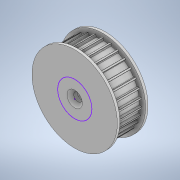
# Autodesk Inventor part: zahnrad
Saved by Autodesk Inventor 2021 (Build 250183000, 183)
## iProperties
Created: 2021-08-02
Part Number: zahnrad
Material: Generisch
Document SubType Name: Modeling
Designer: stroh
Density: 1 g/cm^3
Appearance: Vorgabe
Author: stroh
Autodesk Inventor part; units mm, degrees
ref_plane "YZ Plane" through (0, 0, 0) normal (1, 0, 0) x (0, 1, 0)
ref_plane "XZ Plane" through (0, 0, 0) normal (0, 1, 0) x (-1, 0, 0)
ref_plane "XY Plane" through (0, 0, 0) normal (0, 0, 1) x (1, 0, 0)
sketch "Skizze1" plane through (0, 0, 0) normal (0, 0, 1) x (1, 0, 0)
  line L0 (-32.159, 0) -> (32.1594, 0) projected
  line L1 (0, -33.3687) -> (0, 39.89) projected
  circle A0 centre (0, 0) radius 21.4859
  line L2 (0, 21.3008) -> (0, 29.4245) construction
  line L3 (0.5, 21.4801) -> (-0.5, 21.4801)
  line L4 (-0.4048, 22.9801) -> (0.395, 22.9801)
  line L5 (-0.5, 22.8801) -> (-0.5, 21.4801)
  line L6 (0.395, 22.9801) -> (0.5, 22.8801)
  line L7 (-0.4048, 22.9801) -> (-0.5, 22.8801)
  line L8 (0.5, 22.8801) -> (0.5, 21.4801)
  line L9 (-4.116, 22.5124) -> (-3.8341, 21.141)
  line L10 (-4.239, 22.5892) -> (-4.116, 22.5124)
  line L11 (-5.0223, 22.4282) -> (-4.239, 22.5892)
  line L12 (-5.0223, 22.4282) -> (-5.0955, 22.3111)
  line L13 (-5.0955, 22.3111) -> (-4.8137, 20.9398)
  line L14 (-3.8341, 21.141) -> (-4.8137, 20.9398)
  line L15 (-8.5634, 21.223) -> (-8.0113, 19.9365)
  line L16 (-8.6994, 21.2735) -> (-8.5634, 21.223)
  line L17 (-9.4343, 20.9581) -> (-8.6994, 21.2735)
  line L18 (-9.4343, 20.9581) -> (-9.4824, 20.8287)
  line L19 (-9.4824, 20.8287) -> (-8.9303, 19.5421)
  line L20 (-8.0113, 19.9365) -> (-8.9303, 19.5421)
  line L21 (-12.6603, 19.0648) -> (-11.8605, 17.9157)
  line L22 (-12.8036, 19.0869) -> (-12.6603, 19.0648)
  line L23 (-13.46, 18.63) -> (-12.8036, 19.0869)
  line L24 (-13.46, 18.63) -> (-13.4811, 18.4935)
  line L25 (-13.4811, 18.4935) -> (-12.6813, 17.3444)
  line L26 (-11.8605, 17.9157) -> (-12.6813, 17.3444)
  line L27 (-16.2388, 16.126) -> (-15.2241, 15.1615)
  line L28 (-16.3837, 16.1188) -> (-16.2388, 16.126)
  line L29 (-16.9347, 15.5392) -> (-16.3837, 16.1188)
  line L30 (-16.9347, 15.5392) -> (-16.9278, 15.4012)
  line L31 (-16.9278, 15.4012) -> (-15.9131, 14.4367)
  line L32 (-15.2241, 15.1615) -> (-15.9131, 14.4367)
  line L33 (-19.1526, 12.5271) -> (-17.9645, 11.7865)
  line L34 (-19.293, 12.4908) -> (-19.1526, 12.5271)
  line L35 (-19.716, 11.8121) -> (-19.293, 12.4908)
  line L36 (-19.716, 11.8121) -> (-19.6815, 11.6784)
  line L37 (-19.6815, 11.6784) -> (-18.4934, 10.9379)
  line L38 (-17.9645, 11.7865) -> (-18.4934, 10.9379)
  line L39 (-21.2822, 8.4153) -> (-19.9694, 7.929)
  line L40 (-21.4125, 8.3515) -> (-21.2822, 8.4153)
  line L41 (-21.6902, 7.6015) -> (-21.4125, 8.3515)
  line L42 (-21.6902, 7.6015) -> (-21.6295, 7.4775)
  line L43 (-21.6295, 7.4775) -> (-20.3167, 6.9913)
  line L44 (-19.9694, 7.929) -> (-20.3167, 6.9913)
  line L45 (-22.5405, 3.9589) -> (-21.1567, 3.7469)
  line L46 (-22.6553, 3.8703) -> (-22.5405, 3.9589)
  line L47 (-22.7764, 3.0797) -> (-22.6553, 3.8703)
  line L48 (-22.7764, 3.0797) -> (-22.692, 2.9704)
  line L49 (-22.692, 2.9704) -> (-21.3081, 2.7584)
  line L50 (-21.1567, 3.7469) -> (-21.3081, 2.7584)
  line L51 (-22.8761, -0.6595) -> (-21.4779, -0.5886)
  line L52 (-22.9706, -0.7694) -> (-22.8761, -0.6595)
  line L53 (-22.9301, -1.5682) -> (-22.9706, -0.7694)
  line L54 (-22.9301, -1.5682) -> (-22.8254, -1.6582)
  line L55 (-22.8254, -1.6582) -> (-21.4272, -1.5873)
  line L56 (-21.4779, -0.5886) -> (-21.4272, -1.5873)
  line L57 (-22.275, -5.2509) -> (-20.9197, -4.9)
  line L58 (-22.3455, -5.3776) -> (-22.275, -5.2509)
  line L59 (-22.1451, -6.1519) -> (-22.3455, -5.3776)
  line L60 (-22.1451, -6.1519) -> (-22.0244, -6.219)
  line L61 (-22.0244, -6.219) -> (-20.6691, -5.8681)
  line L62 (-20.9197, -4.9) -> (-20.6691, -5.8681)
  line L63 (-20.7621, -9.6274) -> (-19.5051, -9.0108)
  line L64 (-20.8056, -9.7657) -> (-20.7621, -9.6274)
  line L65 (-20.4534, -10.4837) -> (-20.8056, -9.7657)
  line L66 (-20.4534, -10.4837) -> (-20.3217, -10.5252)
  line L67 (-20.3217, -10.5252) -> (-19.0647, -9.9086)
  line L68 (-19.5051, -9.0108) -> (-19.0647, -9.9086)
  line L69 (-18.3991, -13.6097) -> (-17.292, -12.7527)
  line L70 (-18.4139, -13.7539) -> (-18.3991, -13.6097)
  line L71 (-17.9243, -14.3863) -> (-18.4139, -13.7539)
  line L72 (-17.9243, -14.3863) -> (-17.787, -14.4004)
  line L73 (-17.787, -14.4004) -> (-16.6799, -13.5435)
  line L74 (-17.292, -12.7527) -> (-16.6799, -13.5435)
  line L75 (-15.2828, -17.0348) -> (-14.3709, -15.9725)
  line L76 (-15.2683, -17.1791) -> (-15.2828, -17.0348)
  line L77 (-14.6615, -17.7) -> (-15.2683, -17.1791)
  line L78 (-14.6615, -17.7) -> (-14.5241, -17.6861)
  line L79 (-14.5241, -17.6861) -> (-13.6122, -16.6239)
  line L80 (-14.3709, -15.9725) -> (-13.6122, -16.6239)
  line L81 (-11.5409, -19.7625) -> (-10.8615, -18.5384)
  line L82 (-11.4976, -19.9009) -> (-11.5409, -19.7625)
  line L83 (-10.7984, -20.289) -> (-11.4976, -19.9009)
  line L84 (-10.7984, -20.289) -> (-10.6666, -20.2478)
  line L85 (-10.6666, -20.2478) -> (-9.9872, -19.0237)
  line L86 (-10.8615, -18.5384) -> (-9.9872, -19.0237)
  line L87 (-7.3265, -21.6811) -> (-6.9074, -20.3453)
  line L88 (-7.2563, -21.808) -> (-7.3265, -21.6811)
  line L89 (-6.4932, -22.0474) -> (-7.2563, -21.808)
  line L90 (-6.4932, -22.0474) -> (-6.3724, -21.9805)
  line L91 (-6.3724, -21.9805) -> (-5.9533, -20.6447)
  line L92 (-6.9074, -20.3453) -> (-5.9533, -20.6447)
  line L93 (-2.8122, -22.7121) -> (-2.6705, -21.3193)
  line L94 (-2.7178, -22.8222) -> (-2.8122, -22.7121)
  line L95 (-1.9222, -22.9031) -> (-2.7178, -22.8222)
  line L96 (-1.9222, -22.9031) -> (-1.8173, -22.8133)
  line L97 (-1.8173, -22.8133) -> (-1.6757, -21.4205)
  line L98 (-2.6705, -21.3193) -> (-1.6757, -21.4205)
  line L99 (1.8173, -22.8133) -> (1.6757, -21.4205)
  line L100 (1.9319, -22.9022) -> (1.8173, -22.8133)
  line L101 (2.7276, -22.8212) -> (1.9319, -22.9022)
  line L102 (2.7276, -22.8212) -> (2.8122, -22.7121)
  line L103 (2.8122, -22.7121) -> (2.6705, -21.3193)
  line L104 (1.6757, -21.4205) -> (2.6705, -21.3193)
  line L105 (6.3724, -21.9805) -> (5.9533, -20.6447)
  line L106 (6.5025, -22.0445) -> (6.3724, -21.9805)
  line L107 (7.2656, -21.805) -> (6.5025, -22.0445)
  line L108 (7.2656, -21.805) -> (7.3265, -21.6811)
  line L109 (7.3265, -21.6811) -> (6.9074, -20.3453)
  line L110 (5.9533, -20.6447) -> (6.9074, -20.3453)
  line L111 (10.6666, -20.2478) -> (9.9872, -19.0237)
  line L112 (10.8069, -20.2843) -> (10.6666, -20.2478)
  line L113 (11.5062, -19.8961) -> (10.8069, -20.2843)
  line L114 (11.5062, -19.8961) -> (11.5409, -19.7625)
  line L115 (11.5409, -19.7625) -> (10.8615, -18.5384)
  line L116 (9.9872, -19.0237) -> (10.8615, -18.5384)
  line L117 (14.5241, -17.6861) -> (13.6122, -16.6239)
  line L118 (14.6689, -17.6936) -> (14.5241, -17.6861)
  line L119 (15.2757, -17.1727) -> (14.6689, -17.6936)
  line L120 (15.2757, -17.1727) -> (15.2828, -17.0348)
  line L121 (15.2828, -17.0348) -> (14.3709, -15.9725)
  line L122 (13.6122, -16.6239) -> (14.3709, -15.9725)
  line L123 (17.787, -14.4004) -> (16.6799, -13.5435)
  line L124 (17.9303, -14.3786) -> (17.787, -14.4004)
  line L125 (18.4199, -13.7462) -> (17.9303, -14.3786)
  line L126 (18.4199, -13.7462) -> (18.3991, -13.6097)
  line L127 (18.3991, -13.6097) -> (17.292, -12.7527)
  line L128 (16.6799, -13.5435) -> (17.292, -12.7527)
  line L129 (20.3217, -10.5252) -> (19.0647, -9.9086)
  line L130 (20.4577, -10.4749) -> (20.3217, -10.5252)
  line L131 (20.8099, -9.7569) -> (20.4577, -10.4749)
  line L132 (20.8099, -9.7569) -> (20.7621, -9.6274)
  line L133 (20.7621, -9.6274) -> (19.5051, -9.0108)
  line L134 (19.0647, -9.9086) -> (19.5051, -9.0108)
  line L135 (22.0244, -6.219) -> (20.6691, -5.8681)
  line L136 (22.1475, -6.1424) -> (22.0244, -6.219)
  line L137 (22.348, -5.3682) -> (22.1475, -6.1424)
  line L138 (22.348, -5.3682) -> (22.275, -5.2509)
  line L139 (22.275, -5.2509) -> (20.9197, -4.9)
  line L140 (20.6691, -5.8681) -> (20.9197, -4.9)
  line L141 (22.8254, -1.6582) -> (21.4272, -1.5873)
  line L142 (22.9306, -1.5584) -> (22.8254, -1.6582)
  line L143 (22.9711, -0.7597) -> (22.9306, -1.5584)
  line L144 (22.9711, -0.7597) -> (22.8761, -0.6595)
  line L145 (22.8761, -0.6595) -> (21.4779, -0.5886)
  line L146 (21.4272, -1.5873) -> (21.4779, -0.5886)
  line L147 (22.692, 2.9704) -> (21.3081, 2.7584)
  line L148 (22.7749, 3.0894) -> (22.692, 2.9704)
  line L149 (22.6538, 3.8799) -> (22.7749, 3.0894)
  line L150 (22.6538, 3.8799) -> (22.5405, 3.9589)
  line L151 (22.5405, 3.9589) -> (21.1567, 3.7469)
  line L152 (21.3081, 2.7584) -> (21.1567, 3.7469)
  line L153 (21.6295, 7.4775) -> (20.3167, 6.9913)
  line L154 (21.6868, 7.6107) -> (21.6295, 7.4775)
  line L155 (21.4091, 8.3607) -> (21.6868, 7.6107)
  line L156 (21.4091, 8.3607) -> (21.2822, 8.4153)
  line L157 (21.2822, 8.4153) -> (19.9694, 7.929)
  line L158 (20.3167, 6.9913) -> (19.9694, 7.929)
  line L159 (19.6815, 11.6784) -> (18.4934, 10.9379)
  line L160 (19.7109, 11.8204) -> (19.6815, 11.6784)
  line L161 (19.2878, 12.4992) -> (19.7109, 11.8204)
  line L162 (19.2878, 12.4992) -> (19.1526, 12.5271)
  line L163 (19.1526, 12.5271) -> (17.9645, 11.7865)
  line L164 (18.4934, 10.9379) -> (17.9645, 11.7865)
  line L165 (16.9278, 15.4012) -> (15.9131, 14.4367)
  line L166 (16.9279, 15.5462) -> (16.9278, 15.4012)
  line L167 (16.3769, 16.1259) -> (16.9279, 15.5462)
  line L168 (16.3769, 16.1259) -> (16.2388, 16.126)
  line L169 (16.2388, 16.126) -> (15.2241, 15.1615)
  line L170 (15.9131, 14.4367) -> (15.2241, 15.1615)
  line L171 (13.4811, 18.4935) -> (12.6813, 17.3444)
  line L172 (13.452, 18.6356) -> (13.4811, 18.4935)
  line L173 (12.7956, 19.0925) -> (13.452, 18.6356)
  line L174 (12.7956, 19.0925) -> (12.6603, 19.0648)
  line L175 (12.6603, 19.0648) -> (11.8605, 17.9157)
  line L176 (12.6813, 17.3444) -> (11.8605, 17.9157)
  line L177 (9.4824, 20.8287) -> (8.9303, 19.5421)
  line L178 (9.4253, 20.962) -> (9.4824, 20.8287)
  line L179 (8.6904, 21.2774) -> (9.4253, 20.962)
  line L180 (8.6904, 21.2774) -> (8.5634, 21.223)
  line L181 (8.5634, 21.223) -> (8.0113, 19.9365)
  line L182 (8.9303, 19.5421) -> (8.0113, 19.9365)
  line L183 (5.0955, 22.3111) -> (4.8137, 20.9398)
  line L184 (5.0128, 22.4302) -> (5.0955, 22.3111)
  line L185 (4.2294, 22.5912) -> (5.0128, 22.4302)
  line L186 (4.2294, 22.5912) -> (4.116, 22.5124)
  line L187 (4.116, 22.5124) -> (3.8341, 21.141)
  line L188 (4.8137, 20.9398) -> (3.8341, 21.141)
  point P0 (-21.4859, 0)
  point P1 (21.4859, 0)
  dimension "d0" = 42.9718
  dimension "d2" = 1
  dimension "d4" = 1.5
  dimension "d53" = 0.5
  dimension "d54" = 0.1
  dimension "d56" = 0.1
  dimension "d112" = 360
  constraints: 374 end point, 2 horizontal, 2 point on line, 1 coincident, 1 perpendicular, 1 vertical, 377 other
  measures "d2" distance of L3.start L3.end
  measures "d4" distance between parallel lines of L3 L4
  measures "d53" distance from line of L1 L5.start
  measures "d54" distance from line of L4 L6.end
  measures "d56" distance from line of L5.start L4
extrude "Extrusion1" add sketch "Skizze1" along normal blind 15 contours A0 L50 L44 L38 L32 L26 L20 L14 L3 L1 L0 | L0 L1 A0 L98 L92 L86 L80 L74 L68 L62 L56 | L1 L3 A0 L188 L182 L176 L170 L164 L158 L152 L0 | L0 A0 L146 L140 L134 L128 L122 L116 L110 L104 L1 | A0 L50 | L56 A0 | L3 A0 L1 | L1 A0 L3 | L152 A0 | A0 L146 | A0 L98 | L104 A0 | A0 L44 | L62 A0 | A0 L188 | L14 A0 | L158 A0 | A0 L140 | A0 L92 | L110 A0 | A0 L38 | L68 A0 | A0 L182 | L20 A0 | L164 A0 | A0 L134 | A0 L86 | L116 A0 | A0 L32 | L74 A0 | A0 L176 | L26 A0 | L170 A0 | A0 L128 | A0 L80 | L122 A0
extrude "Extrusion2" add sketch "Skizze1" along normal blind 15
sketch "Skizze2" plane through (0, 0, 15) normal (0, 0, 1) x (1, 0, 0)
  circle A0 centre (0, 0) radius 25
  dimension "d14" = 50
  constraints: 1 centre point, 1 coincident
  measures "d14" diameter of A0
extrude "Extrusion3" add sketch "Skizze2" along normal blind 1.5
sketch "Skizze3" plane through (0, 0, 0) normal (0, 0, -1) x (-1, 0, 0)
  circle A0 centre (0, 0) radius 25
  dimension "d93" = 50
  constraints: 1 centre point, 1 coincident
  measures "d93" diameter of A0
extrude "Extrusion4" add sketch "Skizze3" along normal blind 1.5
sketch "Skizze4" plane through (0, 0, -1.5) normal (0, 0, -1) x (-1, 0, 0)
  circle A0 centre (0, 0) radius 7.5
  dimension "d19" = 15
  constraints: 1 centre point, 1 coincident
  measures "d19" diameter of A0
extrude "Extrusion5" cut sketch "Skizze4" against normal blind 9
sketch "Skizze5" plane through (0, 0, 7.5) normal (0, 0, -1) x (-1, 0, 0)
  line L0 (35, 0) -> (-35, 0) projected
  line L1 (0, -35) -> (0, 35) projected
  line L2 (-6.5054, 0) -> (-4.6, 1.9054)
  line L3 (-1.9054, 4.6) -> (0, 6.5054)
  line L4 (-4.6, 4.6) -> (-1.9054, 4.6)
  line L5 (1.9054, 4.6) -> (4.6, 4.6)
  line L6 (0, 6.5054) -> (1.9054, 4.6)
  line L7 (4.6, 1.9054) -> (6.5054, 0)
  line L8 (4.6, 4.6) -> (4.6, 1.9054)
  line L9 (4.6, -1.9054) -> (4.6, -4.6)
  line L10 (6.5054, 0) -> (4.6, -1.9054)
  line L11 (1.9054, -4.6) -> (0, -6.5054)
  line L12 (4.6, -4.6) -> (1.9054, -4.6)
  line L13 (-1.9054, -4.6) -> (-4.6, -4.6)
  line L14 (0, -6.5054) -> (-1.9054, -4.6)
  line L15 (-4.6, -1.9054) -> (-6.5054, 0)
  line L16 (-4.6, -4.6) -> (-4.6, -1.9054)
  line L17 (-4.6, 1.9054) -> (-4.6, 4.6)
  point P0 (0, 0)
  dimension "d29" = 9.2
  dimension "d30" = 9.2
  constraints: 32 end point, 16 parallel, 8 perpendicular, 2 horizontal, 2 point on line
  measures "d29" distance of L4.start L5.end
  measures "d30" distance of L5.end L9.end
extrude "Extrusion6" cut sketch "Skizze5" against normal blind 5
sketch "Skizze6" plane through (0, 0, 12.5) normal (0, 0, -1) x (-1, 0, 0)
  circle A0 centre (0, 0) radius 2.5
  dimension "d41" = 5
  constraints: 1 centre point, 1 coincident
  measures "d41" diameter of A0
extrude "Extrusion7" cut sketch "Skizze6" against normal blind 5
sketch "Skizze7" plane through (0, 0, -1.5) normal (0, 0, -1) x (-1, 0, 0)
  circle A0 centre (0, 0) radius 2.5 projected
  circle A1 centre (0, 0) radius 10
  circle A2 centre (0, 0) radius 20
  dimension "d44" = 20
  dimension "d45" = 40
  constraints: 2 centre point, 2 coincident
  measures "d44" diameter of A1
  measures "d45" diameter of A2
extrude "Extrusion8" cut sketch "Skizze7" against normal blind 5 contours A2
sketch "Skizze8" plane through (0, 0, 16.5) normal (0, 0, 1) x (1, 0, 0)
  circle A0 centre (0, 0) radius 10
  constraints: 1 centre point
chamfer "Fase1" distance 2 angle 45 1 edges at (2.5, 0, 16.5)
